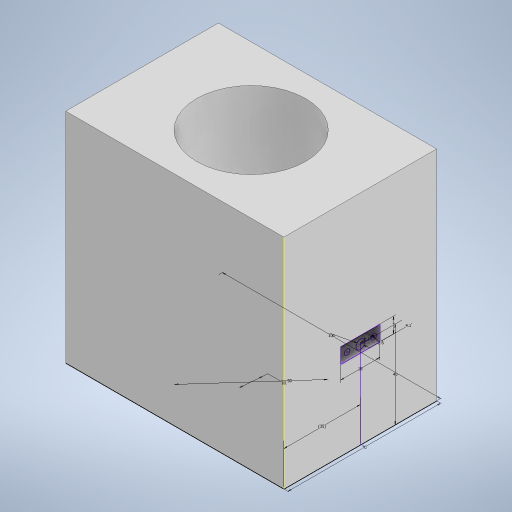
# Autodesk Inventor part: onefour
Saved by Autodesk Inventor 2024 (Build 280153000, 153)
## iProperties
Created: 2024-04-09
Part Number: onefour
Material: 一般
Document SubType Name: Sheet Metal
Designer: QEL
Density: 1 g/cm^3
Sheet Metal Rule: 預設 mm (_M)
Appearance: 預設
Author: QEL
Autodesk Inventor part; units mm, degrees
ref_plane "YZ Plane" through (0, 0, 0) normal (1, 0, 0) x (0, 1, 0)
ref_plane "XZ Plane" through (0, 0, 0) normal (0, 1, 0) x (-1, 0, 0)
ref_plane "XY Plane" through (0, 0, 0) normal (0, 0, 1) x (1, 0, 0)
sketch "草圖1" plane through (0, 0, 0) normal (0, 1, 0) x (-1, 0, 0)
  line L0 (50, 35) -> (-50, 35)
  line L1 (-50, 35) -> (-50, -35)
  line L2 (-50, -35) -> (50, -35)
  line L3 (50, -35) -> (50, 35)
  line L4 (50, 35) -> (-50, -35) construction
  line L5 (-50, 35) -> (50, -35) construction
  circle A0 centre (0, 0) radius 25
  circle A1 centre (0, 0) radius 5
  dimension "d0" = 100
  dimension "d1" = 70
  dimension "d2" = 50
  dimension "d3" = 10
  constraints: 12 end point, 2 centre point, 2 coincident, 2 midpoint, 2 parallel, 1 horizontal, 1 perpendicular
  measures "d0" distance of L2.end L1.end
  measures "d1" distance of L1.end L0.end
  measures "d2" diameter of A0
  measures "d3" diameter of A1
extrude "擠出1" add sketch "草圖1" along normal blind 15 contours A0
extrude "擠出2" add sketch "草圖1" along normal blind 100 contours L3 L2 L1 L0
extrude "擠出3" add sketch "草圖1" along normal blind 34 contours A1
sketch "草圖2" plane through (50, 0, 35) normal (1, 0, 0) x (0, 0, -1)
  line L0 (0, 0) -> (0, 100) projected
  line L1 (0, 0) -> (70, 0) projected
  line L2 (35, 0) -> (35, 40)
  circle A0 centre (35, 40) radius 2.05
  line L3 (26, 43.5) -> (44, 43.5)
  line L4 (44, 43.5) -> (44, 36.5)
  line L5 (44, 36.5) -> (26, 36.5)
  line L6 (26, 36.5) -> (26, 43.5)
  line L7 (26, 43.5) -> (44, 36.5) construction
  line L8 (44, 43.5) -> (26, 36.5) construction
  line L9 (35, 40) -> (41.1, 40)
  circle A1 centre (41.1, 40) radius 1.3
  circle A2 centre (28.9, 40) radius 1.3
  dimension "d10" = 35
  dimension "d11" = 40
  dimension "d12" = 4.1
  dimension "d20" = 18
  dimension "d21" = 7
  dimension "d24" = 6.1
  dimension "d25" = 2.6
  constraints: 16 end point, 3 centre point, 2 coincident, 2 horizontal, 2 midpoint, 2 parallel, 1 perpendicular, 1 symmetric about line, 1 other
  measures "d10" distance of L0.start L2.start
  measures "d11" distance of L2.start L2.end
  measures "d12" diameter of A0
  measures "d20" distance of L4.end L5.end
  measures "d21" distance of L3.end L4.end
  measures "d24" distance of L9.start L9.end
  measures "d25" diameter of A1
hole "孔1" at (50, 40, 0) direction (-1, 0, 0) diameter 4.1 depth 35
extrude "擠出4" cut sketch "草圖2" against normal blind 13 contours L3 L4 L5 L6 | A1 | A2
hole "孔2" at (50, 40, 6.1) at (50, 40, -6.1) direction (-1, 0, 0) diameter 2.1129 depth 20 thread size "M2.6x0.45" class "6H" standard "ANSI Metric M Profile"
equation "\"d27\" = d25"
equation "\"折彎半徑\" = 厚度"
equation "\"折彎離隙寬度\" = 厚度"
equation "\"折彎離隙深度\" = 0.5 * 厚度"
equation "\"轉角離隙大小\" = 4 * 厚度"
equation "\"最小剩餘\" = 2 * 厚度"
equation "\"轉移半徑\" = 折彎半徑"
equation "\"Jacobi半徑大小\" = 折彎半徑"
equation "\"間隙大小\" = 厚度"
equation "\"厚度\" = 0.5"
